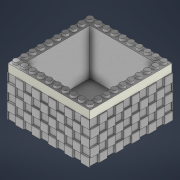
# Autodesk Inventor part: 110033226_ipt_30_城堡四圓塔的頂部
Saved by Autodesk Inventor 2022 (Build 260153000, 153)
## iProperties
Created: 2022-06-24
Part Number: 110033226_ipt_30_城堡四圓塔的頂部
Material: 一般
Document SubType Name: Modeling
Designer: User
Density: 1 g/cm^3
Appearance: 預設
Author: User
Autodesk Inventor part; units mm, degrees
ref_plane "YZ Plane" through (0, 0, 0) normal (1, 0, 0) x (0, 1, 0)
ref_plane "XY Plane" through (0, 0, 0) normal (0, 0, 1) x (1, 0, 0)
sketch "草圖1" plane through (0, 0, 0) normal (0, 1, 0) x (-1, 0, 0)
  line L0 (50, 0) -> (0, 0)
  line L1 (0, 0) -> (0, -50)
  line L2 (0, -50) -> (50, -50)
  line L3 (50, -50) -> (50, 0)
  circle A0 centre (47.5, -2.5) radius 1.7
  circle A1 centre (47.5, -7.5) radius 1.7
  circle A2 centre (47.5, -12.5) radius 1.7
  circle A3 centre (47.5, -17.5) radius 1.7
  circle A4 centre (47.5, -22.5) radius 1.7
  circle A5 centre (47.5, -27.5) radius 1.7
  circle A6 centre (47.5, -32.5) radius 1.7
  circle A7 centre (47.5, -37.5) radius 1.7
  circle A8 centre (47.5, -42.5) radius 1.7
  circle A9 centre (47.5, -47.5) radius 1.7
  circle A10 centre (42.5, -2.5) radius 1.7
  circle A11 centre (42.5, -7.5) radius 1.7
  circle A12 centre (42.5, -12.5) radius 1.7
  circle A13 centre (42.5, -17.5) radius 1.7
  circle A14 centre (42.5, -22.5) radius 1.7
  circle A15 centre (42.5, -27.5) radius 1.7
  circle A16 centre (42.5, -32.5) radius 1.7
  circle A17 centre (42.5, -37.5) radius 1.7
  circle A18 centre (42.5, -42.5) radius 1.7
  circle A19 centre (42.5, -47.5) radius 1.7
  circle A20 centre (37.5, -2.5) radius 1.7
  circle A21 centre (37.5, -7.5) radius 1.7
  circle A22 centre (37.5, -12.5) radius 1.7
  circle A23 centre (37.5, -17.5) radius 1.7
  circle A24 centre (37.5, -22.5) radius 1.7
  circle A25 centre (37.5, -27.5) radius 1.7
  circle A26 centre (37.5, -32.5) radius 1.7
  circle A27 centre (37.5, -37.5) radius 1.7
  circle A28 centre (37.5, -42.5) radius 1.7
  circle A29 centre (37.5, -47.5) radius 1.7
  circle A30 centre (32.5, -2.5) radius 1.7
  circle A31 centre (32.5, -7.5) radius 1.7
  circle A32 centre (32.5, -12.5) radius 1.7
  circle A33 centre (32.5, -17.5) radius 1.7
  circle A34 centre (32.5, -22.5) radius 1.7
  circle A35 centre (32.5, -27.5) radius 1.7
  circle A36 centre (32.5, -32.5) radius 1.7
  circle A37 centre (32.5, -37.5) radius 1.7
  circle A38 centre (32.5, -42.5) radius 1.7
  circle A39 centre (32.5, -47.5) radius 1.7
  circle A40 centre (27.5, -2.5) radius 1.7
  circle A41 centre (27.5, -7.5) radius 1.7
  circle A42 centre (27.5, -12.5) radius 1.7
  circle A43 centre (27.5, -17.5) radius 1.7
  circle A44 centre (27.5, -22.5) radius 1.7
  circle A45 centre (27.5, -27.5) radius 1.7
  circle A46 centre (27.5, -32.5) radius 1.7
  circle A47 centre (27.5, -37.5) radius 1.7
  circle A48 centre (27.5, -42.5) radius 1.7
  circle A49 centre (27.5, -47.5) radius 1.7
  circle A50 centre (22.5, -2.5) radius 1.7
  circle A51 centre (22.5, -7.5) radius 1.7
  circle A52 centre (22.5, -12.5) radius 1.7
  circle A53 centre (22.5, -17.5) radius 1.7
  circle A54 centre (22.5, -22.5) radius 1.7
  circle A55 centre (22.5, -27.5) radius 1.7
  circle A56 centre (22.5, -32.5) radius 1.7
  circle A57 centre (22.5, -37.5) radius 1.7
  circle A58 centre (22.5, -42.5) radius 1.7
  circle A59 centre (22.5, -47.5) radius 1.7
  circle A60 centre (17.5, -2.5) radius 1.7
  circle A61 centre (17.5, -7.5) radius 1.7
  circle A62 centre (17.5, -12.5) radius 1.7
  circle A63 centre (17.5, -17.5) radius 1.7
  circle A64 centre (17.5, -22.5) radius 1.7
  circle A65 centre (17.5, -27.5) radius 1.7
  circle A66 centre (17.5, -32.5) radius 1.7
  circle A67 centre (17.5, -37.5) radius 1.7
  circle A68 centre (17.5, -42.5) radius 1.7
  circle A69 centre (17.5, -47.5) radius 1.7
  circle A70 centre (12.5, -2.5) radius 1.7
  circle A71 centre (12.5, -7.5) radius 1.7
  circle A72 centre (12.5, -12.5) radius 1.7
  circle A73 centre (12.5, -17.5) radius 1.7
  circle A74 centre (12.5, -22.5) radius 1.7
  circle A75 centre (12.5, -27.5) radius 1.7
  circle A76 centre (12.5, -32.5) radius 1.7
  circle A77 centre (12.5, -37.5) radius 1.7
  circle A78 centre (12.5, -42.5) radius 1.7
  circle A79 centre (12.5, -47.5) radius 1.7
  circle A80 centre (7.5, -2.5) radius 1.7
  circle A81 centre (7.5, -7.5) radius 1.7
  circle A82 centre (7.5, -12.5) radius 1.7
  circle A83 centre (7.5, -17.5) radius 1.7
  circle A84 centre (7.5, -22.5) radius 1.7
  circle A85 centre (7.5, -27.5) radius 1.7
  circle A86 centre (7.5, -32.5) radius 1.7
  circle A87 centre (7.5, -37.5) radius 1.7
  circle A88 centre (7.5, -42.5) radius 1.7
  circle A89 centre (7.5, -47.5) radius 1.7
  circle A90 centre (2.5, -2.5) radius 1.7
  circle A91 centre (2.5, -7.5) radius 1.7
  circle A92 centre (2.5, -12.5) radius 1.7
  circle A93 centre (2.5, -17.5) radius 1.7
  circle A94 centre (2.5, -22.5) radius 1.7
  circle A95 centre (2.5, -27.5) radius 1.7
  circle A96 centre (2.5, -32.5) radius 1.7
  circle A97 centre (2.5, -37.5) radius 1.7
  circle A98 centre (2.5, -42.5) radius 1.7
  circle A99 centre (2.5, -47.5) radius 1.7
  line L4 (40, -10) -> (10, -10)
  line L5 (10, -10) -> (10, -40)
  line L6 (10, -40) -> (40, -40)
  line L7 (40, -40) -> (40, -10)
  dimension "d0" = 50
  dimension "d1" = 50
  dimension "d2" = 3.4
  dimension "d3" = 2.5
  dimension "d4" = 2.5
  dimension "d7" = 5
  dimension "d10" = 5
  dimension "d13" = 10
  constraints: 100 centre point, 16 end point, 4 parallel, 2 horizontal, 2 perpendicular, 1 coincident, 1 vertical, 201 other
  measures "d0" distance of L2.end L1.end
  measures "d1" distance of L1.end L0.end
  measures "d2" diameter of A0
  measures "d3" distance from line of L3 A0.centre
  measures "d4" distance from line of L0 A0.centre
  measures "d7" distance of A0.centre A1.centre
  measures "d10" distance of A0.centre A10.centre
  measures "d13" distance between parallel lines of L3 L7
ref_plane "工作平面1" through (0, 30, 0) normal (0, 1, 0) x (-1, 0, 0)
sketch "草圖2" plane through (0, 30, 0) normal (0, 1, 0) x (-1, 0, 0)
  line L0 (50, -50) -> (50, 0) projected
  line L1 (50, 0) -> (0, 0) projected
  line L2 (0, -50) -> (50, -50) projected
  line L3 (40, -40) -> (40, -10) projected
  line L4 (10, -40) -> (40, -40) projected
  line L5 (40, -10) -> (10, -10) projected
  line L6 (10, -10) -> (10, -40) projected
  line L7 (0, 0) -> (0, -50) projected
  line L8 (45, -5) -> (45, -45)
  line L9 (45, -45) -> (5, -45)
  line L10 (5, -45) -> (5, -5)
  line L11 (5, -5) -> (45, -5)
  dimension "d15" = 5
  constraints: 8 end point, 3 other
  measures "d15" distance between parallel lines of L0 L8
extrude "擠出1" add sketch "草圖2" against normal blind 30 contours L2 L7 L1 L0
extrude "擠出2" add sketch "草圖1" along normal blind 2 contours L3 L2 L1 L0 | A11 | A12 | A13 | A14 | A15 | A16 | A17 | A18 | A21 | A22 | A23 | A24 | A25 | A26 | A27 | A28 | A31 | A32 | A33 | A34 | A35 | A36 | A37 | A38 | A41 | A42 | A43 | A44 | A45 | A46 | A47 | A48 | A51 | A52 | A53 | A54 | A55 | A56 | A57 | A58 | A61 | A62 | A63 | A64 | A65 | A66 | A67 | A68 | A71 | A72 | A73 | A74 | A75 | A76 | A77 | A78 | A81 | A82 | A83 | A84 | A85 | A86 | A87 | A88 | L7 L6 L5 L4
extrude "擠出3" cut sketch "草圖1" along normal blind 1.5 contours A0 | A1 | A2 | A3 | A4 | A5 | A6 | A7 | A8 | A9 | A10 | A11 | A12 | A13 | A14 | A15 | A16 | A17 | A18 | A19 | A20 | A21 | A28 | A29 | A30 | A31 | A38 | A39 | A40 | A41 | A48 | A49 | A50 | A51 | A58 | A59 | A60 | A61 | A68 | A69 | A70 | A71 | A78 | A79 | A80 | A81 | A82 | A83 | A84 | A85 | A86 | A87 | A88 | A89 | A90 | A91 | A92 | A93 | A94 | A95 | A96 | A97 | A98 | A99
sketch "草圖3" plane through (0, 30, 0) normal (0, 1, 0) x (1, 0, 0)
  circle A0 centre (-2.5, 2.5) radius 1.7 projected
  point P0 (0, 0)
extrude "擠出4" add sketch "草圖3" along normal blind 1.5
pattern_linear "矩形陣列1" count 10 spacing 5 along (-1, 0, 0) count 2 spacing 45 along (0, 0, -1) of "擠出4"
pattern_linear "矩形陣列2" count 9 spacing 5 along (0, 0, -1) count 2 spacing 45 along (-1, 0, 0) of "擠出4"
sketch "草圖4" plane through (0, 30, 0) normal (1, 0, 0) x (0, 0, -1)
  line L0 (50, 0) -> (50, -30) projected
  line L1 (50, -30) -> (0, -30) projected
  line L2 (0, -30) -> (0, 0) projected
  line L3 (0, 0) -> (50, 0) projected
  line L4 (0, 0) -> (50, 0)
  line L5 (0, 0) -> (0, -30)
  line L6 (4.2, -30) -> (0.8, -30) projected
  line L7 (5, 0) -> (5, -30)
  line L8 (10, 0) -> (10, -30)
  line L9 (15, 0) -> (15, -30)
  line L10 (20, 0) -> (20, -30)
  line L11 (25, 0) -> (25, -30)
  line L12 (30, 0) -> (30, -30)
  line L13 (35, 0) -> (35, -30)
  line L14 (40, 0) -> (40, -30)
  line L15 (45, 0) -> (45, -30)
  line L16 (0, -5) -> (50, -5)
  line L17 (0, -10) -> (50, -10)
  line L18 (0, -15) -> (50, -15)
  line L19 (0, -20) -> (50, -20)
  line L20 (0, -25) -> (50, -25)
  line L21 (0, -30) -> (50, -30)
  point P0 (45, -25)
  point P1 (40, -25)
  point P2 (35, -25)
  point P3 (30, -25)
  point P4 (25, -25)
  point P5 (20, -25)
  point P6 (15, -25)
  point P7 (10, -25)
  point P8 (5, -25)
  point P9 (45, -20)
  point P10 (40, -20)
  point P11 (35, -20)
  point P12 (30, -20)
  point P13 (25, -20)
  point P14 (20, -20)
  point P15 (15, -20)
  point P16 (10, -20)
  point P17 (5, -20)
  point P18 (45, -15)
  point P19 (40, -15)
  point P20 (35, -15)
  point P21 (30, -15)
  point P22 (25, -15)
  point P23 (20, -15)
  point P24 (15, -15)
  point P25 (10, -15)
  point P26 (5, -15)
  point P27 (45, -10)
  point P28 (40, -10)
  point P29 (35, -10)
  point P30 (30, -10)
  point P31 (25, -10)
  point P32 (20, -10)
  point P33 (15, -10)
  point P34 (10, -10)
  point P35 (5, -10)
  point P36 (45, -5)
  point P37 (40, -5)
  point P38 (35, -5)
  point P39 (30, -5)
  point P40 (25, -5)
  point P41 (20, -5)
  point P42 (15, -5)
  point P43 (10, -5)
  point P44 (5, -5)
  dimension "d38" = 5
  dimension "d48" = 5
  constraints: 34 end point, 2 horizontal, 1 perpendicular, 1 vertical, 45 other
  measures "d38" distance of L2.end L7.start
  measures "d48" distance of L2.end L16.start
extrude "擠出5" add sketch "草圖4" along normal blind 0.5 contours L0 L17 L15 L16 | L0 L19 L15 L18 | L15 L18 L14 L17 | L14 L17 L13 L16 | L0 L1 L15 L20 | L15 L20 L14 L19 | L14 L19 L13 L18 | L13 L18 L12 L17 | L12 L17 L11 L16 | L14 L1 L13 L20 | L13 L20 L12 L19 | L12 L19 L11 L18 | L11 L18 L10 L17 | L10 L17 L9 L16 | L12 L1 L11 L20 | L11 L20 L10 L19 | L10 L19 L9 L18 | L9 L18 L8 L17 | L8 L17 L7 L16 | L10 L1 L9 L20 | L9 L20 L8 L19 | L8 L19 L7 L18 | L7 L18 L2 L17 | L8 L1 L7 L20 | L7 L20 L2 L19
extrude "擠出6" cut sketch "草圖4" against normal blind 0.5 contours L0 L18 L15 L17 | L15 L17 L14 L16 | L0 L20 L15 L19 | L15 L19 L14 L18 | L14 L18 L13 L17 | L13 L17 L12 L16 | L15 L1 L14 L20 | L14 L20 L13 L19 | L13 L19 L12 L18 | L12 L18 L11 L17 | L11 L17 L10 L16 | L13 L1 L12 L20 | L12 L20 L11 L19 | L11 L19 L10 L18 | L10 L18 L9 L17 | L9 L17 L8 L16 | L11 L1 L10 L20 | L10 L20 L9 L19 | L9 L19 L8 L18 | L8 L18 L7 L17 | L7 L17 L2 L16 | L9 L1 L8 L20 | L8 L20 L7 L19 | L7 L19 L2 L18 | L7 L1 L2 L20
ref_plane "工作平面2" through (0, 30, -25) normal (0, 0, -1) x (-1, 0, 0)
ref_plane "工作平面3" through (-25, 30, -45) normal (-1, 0, 0) x (0, 0, 1)
pattern_circular "環形陣列1" count 4 over 360 about axis through (-25, 30, -25) along (0, 1, 0) of "擠出6", "擠出5"
